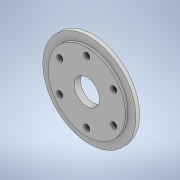
# Autodesk Inventor part: Worm Gear5-Bottom
Saved by Autodesk Inventor 2022.1 (Build 261234000, 234)
## iProperties
Created: 2021-07-06
Part Number: Worm Gear5-Bottom
Material: Generic
Document SubType Name: Modeling
Designer: robst
Density: 1 g/cm^3
Appearance: Default
Author: robst
Autodesk Inventor part; units mm, degrees
ref_plane "YZ Plane" through (0, 0, 0) normal (1, 0, 0) x (0, 1, 0)
ref_plane "XZ Plane" through (0, 0, 0) normal (0, 1, 0) x (-1, 0, 0)
ref_plane "XY Plane" through (0, 0, 0) normal (0, 0, 1) x (1, 0, 0)
sketch "Sketch1" plane through (0, 0, 0) normal (0, 0, 1) x (1, 0, 0)
  circle A0 centre (0, 0) radius 12.8905
  circle A1 centre (0, 0) radius 47.4345
  dimension "d0" = 25.781
  dimension "d1" = 94.869
  constraints: 2 centre point, 2 coincident
  measures "d0" diameter of A0
  measures "d1" diameter of A1
extrude "Extrusion1" add sketch "Sketch1" along normal blind 3.81
sketch "Sketch2" plane through (0, 0, 3.81) normal (0, 0, 1) x (1, 0, 0)
  circle A0 centre (0, 0) radius 12.8905
  circle A1 centre (0, 0) radius 39.37
  dimension "d4" = 78.74
  constraints: 2 centre point, 2 coincident
  measures "d4" diameter of A1
extrude "Extrusion2" add sketch "Sketch2" along normal blind 2.54
sketch "Sketch4" plane through (0, 0, 6.35) normal (0, 0, 1) x (1, 0, 0)
  point P0 (0, 0)
  point P1 (0, 31.75)
  point P2 (-27.4963, 15.875)
  point P3 (-27.4963, -15.875)
  point P4 (0, -31.75)
  point P5 (27.4963, -15.875)
  point P6 (27.4963, 15.875)
  dimension "d19" = 31.75
  dimension "d22" = 360
  constraints: 7 other
  measures "d19" distance of point (0, 0) point (0, 31.75)
hole "Hole2" at (0, 31.75, 6.35) at (-27.4963, 15.875, 6.35) at (-27.4963, -15.875, 6.35) at (0, -31.75, 6.35) at (27.4963, -15.875, 6.35) at (27.4963, 15.875, 6.35) direction (0, 0, -1) diameter 5.5372 depth 6.35 tip angle 118 counterbore diameter 6.3246 counterbore depth 4.9378
body "Solid1"
